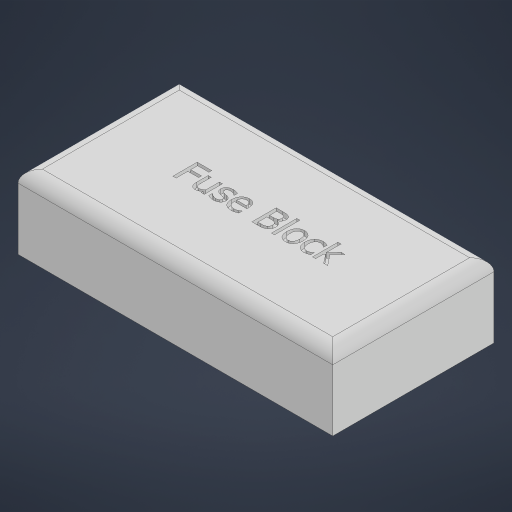
# Autodesk Inventor part: FuseBlock
Saved by Autodesk Inventor 2023 (Build 270158000, 158)
## iProperties
Created: 2023-01-24
Part Number: FuseBlock
Material: Generic
Document SubType Name: Modeling
Designer: Nebil
Density: 1 g/cm^3
Appearance: Default
Author: Nebil
Autodesk Inventor part; units mm, degrees
ref_plane "YZ Plane" through (0, 0, 0) normal (1, 0, 0) x (0, 1, 0)
ref_plane "XZ Plane" through (0, 0, 0) normal (0, 1, 0) x (-1, 0, 0)
ref_plane "XY Plane" through (0, 0, 0) normal (0, 0, 1) x (1, 0, 0)
sketch "Sketch1" plane through (0, 0, 0) normal (0, 1, 0) x (-1, 0, 0)
  line L0 (-82.1944, 42.1005) -> (82.1944, 42.1005)
  line L1 (82.1944, 42.1005) -> (82.1944, -42.1005)
  line L2 (82.1944, -42.1005) -> (-82.1944, -42.1005)
  line L3 (-82.1944, -42.1005) -> (-82.1944, 42.1005)
  line L4 (-82.1944, 42.1005) -> (82.1944, -42.1005) construction
  line L5 (82.1944, 42.1005) -> (-82.1944, -42.1005) construction
  point P0 (0, 0)
  dimension "d0" = 84.201
  dimension "d1" = 164.3888
  constraints: 12 end point, 2 midpoint, 2 parallel, 1 horizontal, 1 perpendicular
  measures "d0" distance of L0.end L1.end
  measures "d1" distance of L1.end L2.end
extrude "Extrusion1" add sketch "Sketch1" along normal blind 38.5572
fillet "Fillet1" radius 6.35 4 edges at (0, 38.5572, 42.1005) (82.1944, 38.5572, 0) (0, 38.5572, -42.1005) (-82.1944, 38.5572, 0)
sketch "Sketch2" plane through (0, 38.5572, 0) normal (0, 1, 0) x (1, 0, 0)
  line L0 (-39.8215, 8.3835) -> (450.9707, 8.3835) construction
  line L1 (450.9707, 8.3835) -> (450.9707, -72.8183) construction
  line L2 (450.9707, -72.8183) -> (-39.8215, -72.8183) construction
  line L3 (-39.8215, -72.8183) -> (-39.8215, 8.3835) construction
  line L4 (-30.9397, 6.3148) -> (-36.8472, 6.3148)
  line L5 (-36.8472, 6.3148) -> (-36.8472, 2.7333)
  line L6 (-36.8472, 2.7333) -> (-31.1867, 2.7333)
  line L7 (-31.1867, 2.7333) -> (-31.1867, 1.2307)
  line L8 (-31.1867, 1.2307) -> (-36.8472, 1.2307)
  line L9 (-36.8472, 1.2307) -> (-36.8472, -4.8826)
  line L10 (-36.8472, -4.8826) -> (-38.535, -4.8826)
  line L11 (-38.535, -4.8826) -> (-38.535, 7.8174)
  line L12 (-38.535, 7.8174) -> (-30.9397, 7.8174)
  line L13 (-30.9397, 7.8174) -> (-30.9397, 6.3148)
  line L14 (-22.1403, -4.8826) -> (-23.7458, -4.8826)
  line L15 (-23.7458, -4.8826) -> (-23.7458, -3.8328)
  spline S0 degree 2 poles (-23.7458, -3.8328) (-24.4868, -4.4812) (-25.8144, -5.1502) (-26.6378, -5.1502) knots 0 0 0 1 2 2 2
  spline S1 degree 2 poles (-26.6378, -5.1502) (-27.2553, -5.1502) (-28.3565, -4.7385) (-28.7579, -4.2959) knots 0 0 0 1 2 2 2
  spline S2 degree 2 poles (-28.7579, -4.2959) (-29.1695, -3.8534) (-29.6224, -2.5052) (-29.6224, -1.5378) knots 0 0 0 1 2 2 2
  line L16 (-29.6224, -1.5378) -> (-29.6224, 4.6476)
  line L17 (-29.6224, 4.6476) -> (-28.0169, 4.6476)
  line L18 (-28.0169, 4.6476) -> (-28.0169, -0.7865)
  spline S3 degree 2 poles (-28.0169, -0.7865) (-28.0169, -1.5481) (-27.9037, -2.5464) (-27.7081, -2.9169) knots 0 0 0 1 2 2 2
  spline S4 degree 2 poles (-27.7081, -2.9169) (-27.5126, -3.2874) (-26.8436, -3.627) (-26.2158, -3.627) knots 0 0 0 1 2 2 2
  spline S5 degree 2 poles (-26.2158, -3.627) (-25.6292, -3.627) (-24.3015, -2.958) (-23.7458, -2.4743) knots 0 0 0 1 2 2 2
  line L19 (-23.7458, -2.4743) -> (-23.7458, 4.6476)
  line L20 (-23.7458, 4.6476) -> (-22.1403, 4.6476)
  line L21 (-22.1403, 4.6476) -> (-22.1403, -4.8826)
  spline S6 degree 2 poles (-17.2414, -5.109) (-18.1986, -5.109) (-19.8555, -4.5944) (-20.401, -4.3062) knots 0 0 0 1 2 2 2
  line L22 (-20.401, -4.3062) -> (-20.401, -2.5052)
  line L23 (-20.401, -2.5052) -> (-20.3186, -2.5052)
  spline S7 degree 2 poles (-20.3186, -2.5052) (-20.1128, -2.6699) (-19.5571, -3.0609) (-19.0939, -3.2771) knots 0 0 0 1 2 2 2
  spline S8 degree 2 poles (-19.0939, -3.2771) (-18.6926, -3.4726) (-17.7045, -3.7608) (-17.1797, -3.7608) knots 0 0 0 1 2 2 2
  spline S9 degree 2 poles (-17.1797, -3.7608) (-16.7989, -3.7608) (-15.9241, -3.5858) (-15.7182, -3.4417) knots 0 0 0 1 2 2 2
  spline S10 degree 2 poles (-15.7182, -3.4417) (-15.4198, -3.2462) (-15.1522, -2.8036) (-15.1522, -2.3508) knots 0 0 0 1 2 2 2
  spline S11 degree 2 poles (-15.1522, -2.3508) (-15.1522, -1.7848) (-15.7697, -1.1981) (-16.5622, -1.0026) knots 0 0 0 1 2 2 2
  spline S12 degree 2 poles (-16.5622, -1.0026) (-16.8709, -0.9305) (-17.8589, -0.7247) (-18.2809, -0.6115) knots 0 0 0 1 2 2 2
  spline S13 degree 2 poles (-18.2809, -0.6115) (-19.3718, -0.2925) (-20.3598, 1.0249) (-20.3598, 1.9614) knots 0 0 0 1 2 2 2
  spline S14 degree 2 poles (-20.3598, 1.9614) (-20.3598, 3.2582) (-18.4147, 4.874) (-16.8092, 4.874) knots 0 0 0 1 2 2 2
  spline S15 degree 2 poles (-16.8092, 4.874) (-16.0167, 4.874) (-14.4112, 4.4829) (-13.8657, 4.1844) knots 0 0 0 1 2 2 2
  line L24 (-13.8657, 4.1844) -> (-13.8657, 2.4657)
  line L25 (-13.8657, 2.4657) -> (-13.9481, 2.4657)
  spline S16 degree 2 poles (-13.9481, 2.4657) (-14.5656, 2.9597) (-16.0682, 3.5258) (-16.84, 3.5258) knots 0 0 0 1 2 2 2
  spline S17 degree 2 poles (-16.84, 3.5258) (-17.6325, 3.5258) (-18.7234, 2.8568) (-18.7234, 2.1878) knots 0 0 0 1 2 2 2
  spline S18 degree 2 poles (-18.7234, 2.1878) (-18.7234, 1.5806) (-18.0751, 0.994) (-17.3546, 0.8088) knots 0 0 0 1 2 2 2
  spline S19 degree 2 poles (-17.3546, 0.8088) (-17.0047, 0.7161) (-16.1196, 0.5309) (-15.6359, 0.4177) knots 0 0 0 1 2 2 2
  spline S20 degree 2 poles (-15.6359, 0.4177) (-14.5862, 0.1501) (-13.5158, -1.0746) (-13.5158, -2.1347) knots 0 0 0 1 2 2 2
  spline S21 degree 2 poles (-13.5158, -2.1347) (-13.5158, -2.7522) (-13.9995, -3.8431) (-14.4729, -4.2445) knots 0 0 0 1 2 2 2
  spline S22 degree 2 poles (-14.4729, -4.2445) (-14.9772, -4.6664) (-16.2637, -5.109) (-17.2414, -5.109) knots 0 0 0 1 2 2 2
  spline S23 degree 2 poles (-7.8862, -5.0987) (-10.171, -5.0987) (-12.6822, -2.5361) (-12.6822, -0.169) knots 0 0 0 1 2 2 2
  spline S24 degree 2 poles (-12.6822, -0.169) (-12.6822, 2.157) (-10.243, 4.9152) (-8.2773, 4.9152) knots 0 0 0 1 2 2 2
  spline S25 degree 2 poles (-8.2773, 4.9152) (-7.3922, 4.9152) (-6.0234, 4.4006) (-5.5191, 3.8551) knots 0 0 0 1 2 2 2
  spline S26 degree 2 poles (-5.5191, 3.8551) (-5.0045, 3.3096) (-4.4591, 1.735) (-4.4591, 0.5926) knots 0 0 0 1 2 2 2
  line L26 (-4.4591, 0.5926) -> (-4.4591, -0.2822)
  line L27 (-4.4591, -0.2822) -> (-11.0561, -0.2822)
  spline S27 degree 2 poles (-11.0561, -0.2822) (-11.0561, -1.9391) (-9.3888, -3.699) (-7.9068, -3.699) knots 0 0 0 1 2 2 2
  spline S28 degree 2 poles (-7.9068, -3.699) (-7.3819, -3.699) (-6.3631, -3.4623) (-5.9514, -3.2771) knots 0 0 0 1 2 2 2
  spline S29 degree 2 poles (-5.9514, -3.2771) (-5.5191, -3.0712) (-4.9222, -2.711) (-4.7267, -2.5464) knots 0 0 0 1 2 2 2
  line L28 (-4.7267, -2.5464) -> (-4.634, -2.5464)
  line L29 (-4.634, -2.5464) -> (-4.634, -4.2959)
  spline S30 degree 2 poles (-4.634, -4.2959) (-4.9119, -4.4092) (-5.7558, -4.7385) (-6.0852, -4.8311) knots 0 0 0 1 2 2 2
  spline S31 degree 2 poles (-6.0852, -4.8311) (-6.5483, -4.9649) (-7.3099, -5.0987) (-7.8862, -5.0987) knots 0 0 0 1 2 2 2
  spline S32 degree 2 poles (-6.0234, 0.9425) (-6.044, 1.5909) (-6.3116, 2.5378) (-6.5689, 2.8568) knots 0 0 0 1 2 2 2
  spline S33 degree 2 poles (-6.5689, 2.8568) (-6.8468, 3.217) (-7.7216, 3.5978) (-8.3699, 3.5978) knots 0 0 0 1 2 2 2
  spline S34 degree 2 poles (-8.3699, 3.5978) (-9.008, 3.5978) (-9.9034, 3.217) (-10.2739, 2.8465) knots 0 0 0 1 2 2 2
  spline S35 degree 2 poles (-10.2739, 2.8465) (-10.6341, 2.4657) (-11.0046, 1.5498) (-11.0561, 0.9425) knots 0 0 0 1 2 2 2
  line L30 (-11.0561, 0.9425) -> (-6.0234, 0.9425)
  spline S36 degree 2 poles (11.3593, -0.982) (11.3593, -1.9288) (10.6389, -3.38) (10.042, -3.8534) knots 0 0 0 1 2 2 2
  spline S37 degree 2 poles (10.042, -3.8534) (9.3215, -4.4092) (7.6852, -4.8826) (6.3884, -4.8826) knots 0 0 0 1 2 2 2
  line L31 (6.3884, -4.8826) -> (2.7451, -4.8826)
  line L32 (2.7451, -4.8826) -> (2.7451, 7.8174)
  line L33 (2.7451, 7.8174) -> (6.1105, 7.8174)
  spline S38 degree 2 poles (6.1105, 7.8174) (7.469, 7.8174) (8.8275, 7.6425) (9.445, 7.3028) knots 0 0 0 1 2 2 2
  spline S39 degree 2 poles (9.445, 7.3028) (10.1346, 6.9426) (10.7624, 5.7591) (10.7624, 4.9563) knots 0 0 0 1 2 2 2
  spline S40 degree 2 poles (10.7624, 4.9563) (10.7624, 4.0609) (9.8155, 2.6407) (8.9819, 2.2393) knots 0 0 0 1 2 2 2
  line L34 (8.9819, 2.2393) -> (8.9819, 2.1776)
  spline S41 degree 2 poles (8.9819, 2.1776) (10.114, 1.8688) (11.3593, 0.2324) (11.3593, -0.982) knots 0 0 0 1 2 2 2
  spline S42 degree 2 poles (9.5994, -1.054) (9.5994, -0.3336) (9.1878, 0.5926) (8.5702, 0.922) knots 0 0 0 1 2 2 2
  spline S43 degree 2 poles (8.5702, 0.922) (8.1689, 1.1278) (7.222, 1.2513) (6.3472, 1.2513) knots 0 0 0 1 2 2 2
  line L35 (6.3472, 1.2513) -> (4.433, 1.2513)
  line L36 (4.433, 1.2513) -> (4.433, -3.4417)
  line L37 (4.433, -3.4417) -> (5.8018, -3.4417)
  spline S44 degree 2 poles (5.8018, -3.4417) (6.9133, -3.4417) (8.1895, -3.2359) (8.6835, -2.9066) knots 0 0 0 1 2 2 2
  spline S45 degree 2 poles (8.6835, -2.9066) (9.1569, -2.5669) (9.5994, -1.723) (9.5994, -1.054) knots 0 0 0 1 2 2 2
  spline S46 degree 2 poles (9.0025, 4.7196) (9.0025, 5.1724) (8.6938, 5.8517) (8.3541, 6.0472) knots 0 0 0 1 2 2 2
  spline S47 degree 2 poles (8.3541, 6.0472) (7.9425, 6.2737) (6.9442, 6.3766) (6.0488, 6.3766) knots 0 0 0 1 2 2 2
  line L38 (6.0488, 6.3766) -> (4.433, 6.3766)
  line L39 (4.433, 6.3766) -> (4.433, 2.6613)
  line L40 (4.433, 2.6613) -> (6.3472, 2.6613)
  spline S48 degree 2 poles (6.3472, 2.6613) (7.1397, 2.6613) (7.891, 2.8259) (8.2924, 3.0832) knots 0 0 0 1 2 2 2
  spline S49 degree 2 poles (8.2924, 3.0832) (8.6835, 3.3302) (9.0025, 4.1227) (9.0025, 4.7196) knots 0 0 0 1 2 2 2
  line L41 (14.5497, -4.8826) -> (12.9442, -4.8826)
  line L42 (12.9442, -4.8826) -> (12.9442, 8.3835)
  line L43 (12.9442, 8.3835) -> (14.5497, 8.3835)
  line L44 (14.5497, 8.3835) -> (14.5497, -4.8826)
  spline S50 degree 2 poles (24.7386, -0.1175) (24.7386, -2.5258) (22.4229, -5.1502) (20.4881, -5.1502) knots 0 0 0 1 2 2 2
  spline S51 degree 2 poles (20.4881, -5.1502) (18.5018, -5.1502) (16.2273, -2.4434) (16.2273, -0.1175) knots 0 0 0 1 2 2 2
  spline S52 degree 2 poles (16.2273, -0.1175) (16.2273, 2.2702) (18.5738, 4.9152) (20.4881, 4.9152) knots 0 0 0 1 2 2 2
  spline S53 degree 2 poles (20.4881, 4.9152) (22.4229, 4.9152) (24.7386, 2.2805) (24.7386, -0.1175) knots 0 0 0 1 2 2 2
  spline S54 degree 2 poles (23.0816, -0.1175) (23.0816, 1.735) (21.7334, 3.5361) (20.4881, 3.5361) knots 0 0 0 1 2 2 2
  spline S55 degree 2 poles (20.4881, 3.5361) (19.2428, 3.5361) (17.8843, 1.735) (17.8843, -0.1175) knots 0 0 0 1 2 2 2
  spline S56 degree 2 poles (17.8843, -0.1175) (17.8843, -1.9186) (19.2428, -3.7711) (20.4881, -3.7711) knots 0 0 0 1 2 2 2
  spline S57 degree 2 poles (20.4881, -3.7711) (21.7231, -3.7711) (23.0816, -1.9494) (23.0816, -0.1175) knots 0 0 0 1 2 2 2
  spline S58 degree 2 poles (30.1726, -5.0987) (29.1846, -5.0987) (27.5482, -4.4915) (26.9616, -3.874) knots 0 0 0 1 2 2 2
  spline S59 degree 2 poles (26.9616, -3.874) (26.3749, -3.2668) (25.7266, -1.3937) (25.7266, -0.1381) knots 0 0 0 1 2 2 2
  spline S60 degree 2 poles (25.7266, -0.1381) (25.7266, 1.1175) (26.3955, 2.9494) (26.9616, 3.5669) knots 0 0 0 1 2 2 2
  spline S61 degree 2 poles (26.9616, 3.5669) (27.5276, 4.1947) (29.2052, 4.8637) (30.1726, 4.8637) knots 0 0 0 1 2 2 2
  spline S62 degree 2 poles (30.1726, 4.8637) (30.9548, 4.8637) (32.4162, 4.4212) (32.9822, 4.133) knots 0 0 0 1 2 2 2
  line L45 (32.9822, 4.133) -> (32.9822, 2.3319)
  line L46 (32.9822, 2.3319) -> (32.8896, 2.3319)
  spline S63 degree 2 poles (32.8896, 2.3319) (32.7147, 2.476) (32.1795, 2.8465) (31.7987, 3.0421) knots 0 0 0 1 2 2 2
  spline S64 degree 2 poles (31.7987, 3.0421) (31.4591, 3.2067) (30.5534, 3.464) (30.1417, 3.464) knots 0 0 0 1 2 2 2
  spline S65 degree 2 poles (30.1417, 3.464) (28.8964, 3.464) (27.3835, 1.5806) (27.3835, -0.1381) knots 0 0 0 1 2 2 2
  spline S66 degree 2 poles (27.3835, -0.1381) (27.3835, -1.8156) (28.845, -3.699) (30.1417, -3.699) knots 0 0 0 1 2 2 2
  spline S67 degree 2 poles (30.1417, -3.699) (30.9239, -3.699) (32.3442, -3.0506) (32.8896, -2.5464) knots 0 0 0 1 2 2 2
  line L47 (32.8896, -2.5464) -> (32.9822, -2.5464)
  line L48 (32.9822, -2.5464) -> (32.9822, -4.3474)
  spline S68 degree 2 poles (32.9822, -4.3474) (32.7455, -4.4606) (32.0251, -4.7797) (31.7369, -4.8517) knots 0 0 0 1 2 2 2
  spline S69 degree 2 poles (31.7369, -4.8517) (31.3253, -4.9752) (30.6769, -5.0987) (30.1726, -5.0987) knots 0 0 0 1 2 2 2
  line L49 (42.3374, -4.8826) -> (40.2276, -4.8826)
  line L50 (40.2276, -4.8826) -> (36.6873, -0.2822)
  line L51 (36.6873, -0.2822) -> (36.0492, -0.8997)
  line L52 (36.0492, -0.8997) -> (36.0492, -4.8826)
  line L53 (36.0492, -4.8826) -> (34.4437, -4.8826)
  line L54 (34.4437, -4.8826) -> (34.4437, 8.3835)
  line L55 (34.4437, 8.3835) -> (36.0492, 8.3835)
  line L56 (36.0492, 8.3835) -> (36.0492, 0.6235)
  line L57 (36.0492, 0.6235) -> (39.816, 4.6476)
  line L58 (39.816, 4.6476) -> (41.8126, 4.6476)
  line L59 (41.8126, 4.6476) -> (37.9017, 0.6647)
  line L60 (37.9017, 0.6647) -> (42.3374, -4.8826)
  point P0 (0, 0)
  constraints: 2 other
emboss "Emboss1" sketch "Sketch2" operation cut depth 2.54 direction (0, -1, 0)
body "Solid1"
